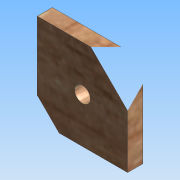
# Autodesk Inventor part: slider_box
Saved by Autodesk Inventor 2015 (Build 190159000, 159)
## iProperties
Created: 2014-09-30
Part Number: slider_box
Material: Wood (Birch)
Document SubType Name: Modeling
Designer: shohei
Density: 0.55 g/cm^3
Appearance: Birch - Natural Polished
Author: shohei
Autodesk Inventor part; units mm, degrees
ref_plane "YZ Plane" through (0, 0, 0) normal (1, 0, 0) x (0, 1, 0)
ref_plane "XZ Plane" through (0, 0, 0) normal (0, 1, 0) x (-1, 0, 0)
ref_plane "XY Plane" through (0, 0, 0) normal (0, 0, 1) x (1, 0, 0)
sketch "Sketch1" plane through (0, 0, 0) normal (0, 1, 0) x (-1, 0, 0)
  line L0 (0, 0) -> (30, 0)
  line L1 (30, 0) -> (30, 30)
  line L2 (30, 30) -> (0, 30)
  line L3 (0, 30) -> (0, 0)
  circle A0 centre (15, 15) radius 2.6
  dimension "d2" = 30
  dimension "d3" = 30
  dimension "d4" = 5.2
  constraints: 8 end point, 2 parallel, 1 centre point, 1 horizontal, 1 perpendicular
  measures "d2" distance of L0.end L1.end
  measures "d3" distance of L1.end L2.end
  measures "d4" diameter of A0
extrude "Extrusion2" add sketch "Sketch1" along normal blind 5
body "Solid2"
